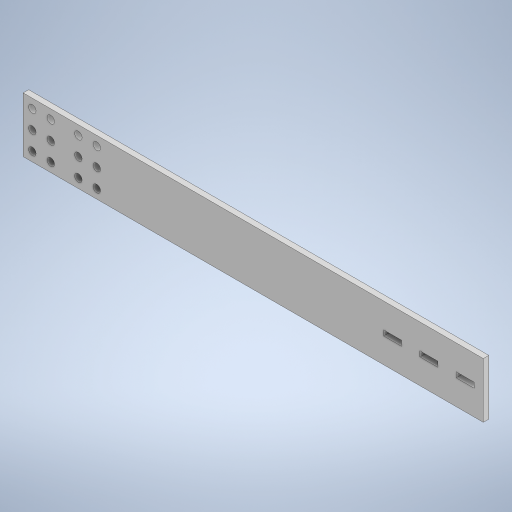
# Autodesk Inventor part: holder_sides
Saved by Autodesk Inventor 2023 (Build 270158000, 158)
## iProperties
Created: 2022-07-08
Part Number: holder_sides
Material: Generic
Document SubType Name: Modeling
Designer: Zayed
Density: 1 g/cm^3
Appearance: Default
Author: Zayed
Autodesk Inventor part; units mm, degrees
ref_plane "YZ Plane" through (0, 0, 0) normal (1, 0, 0) x (0, 1, 0)
ref_plane "XZ Plane" through (0, 0, 0) normal (0, 1, 0) x (-1, 0, 0)
ref_plane "XY Plane" through (0, 0, 0) normal (0, 0, 1) x (1, 0, 0)
sketch "Sketch1" plane through (0, 0, 0) normal (0, 0, 1) x (1, 0, 0)
  line L0 (0, 0) -> (250, 0)
  line L1 (250, 0) -> (250, 30)
  line L2 (-250, -30) -> (250, -30)
  line L3 (250, -30) -> (250, 30)
  line L4 (250, 30) -> (-250, 30)
  line L5 (-250, 30) -> (-250, -30)
  line L6 (-250, -30) -> (250, 30) construction
  line L7 (250, -30) -> (-250, 30) construction
  line L8 (-250, 0) -> (-240, 0)
  line L9 (-240, 0) -> (-240, 20)
  line L10 (-240, 0) -> (-240, -20)
  circle A0 centre (-240, 0) radius 4
  circle A1 centre (-240, 20) radius 4
  circle A2 centre (-240, -20) radius 4
  line L11 (-240, 0) -> (-220, 0)
  line L12 (-220, 0) -> (-220, -20)
  line L13 (-220, 0) -> (-220, 20)
  circle A3 centre (-220, 20) radius 4
  circle A4 centre (-220, 0) radius 4
  circle A5 centre (-220, -20) radius 4
  line L14 (-220, 0) -> (-190, 0)
  line L15 (-190, 0) -> (-190, -20)
  line L16 (-190, 0) -> (-190, 20)
  line L17 (-190, 0) -> (-170, 0)
  line L18 (-170, 0) -> (-170, -20)
  line L19 (-170, 0) -> (-170, 20)
  circle A6 centre (-190, 20) radius 4
  circle A7 centre (-170, 20) radius 4
  circle A8 centre (-170, 0) radius 4
  circle A9 centre (-170, -20) radius 4
  circle A10 centre (-190, 0) radius 4
  circle A11 centre (-190, -20) radius 4
  line L20 (250, 0) -> (240, 0)
  line L21 (240, 0) -> (230.3, 0)
  line L22 (240, 0) -> (240, 2.85)
  line L23 (220.6, -2.85) -> (240, -2.85)
  line L24 (240, -2.85) -> (240, 2.85)
  line L25 (240, 2.85) -> (220.6, 2.85)
  line L26 (220.6, 2.85) -> (220.6, -2.85)
  line L27 (220.6, -2.85) -> (240, 2.85) construction
  line L28 (240, -2.85) -> (220.6, 2.85) construction
  line L29 (220.6, 0) -> (200.6, 0)
  line L30 (200.6, 0) -> (200.6, -2.85)
  line L31 (200.6, 0) -> (190.9, 0)
  line L32 (181.2, 2.85) -> (200.6, 2.85)
  line L33 (200.6, 2.85) -> (200.6, -2.85)
  line L34 (200.6, -2.85) -> (181.2, -2.85)
  line L35 (181.2, -2.85) -> (181.2, 2.85)
  line L36 (181.2, 2.85) -> (200.6, -2.85) construction
  line L37 (200.6, 2.85) -> (181.2, -2.85) construction
  line L38 (181.2, 0) -> (161.2, 0)
  line L39 (161.2, 0) -> (161.2, -2.85)
  line L40 (161.2, 0) -> (151.5, 0)
  line L41 (141.8, 2.85) -> (161.2, 2.85)
  line L42 (161.2, 2.85) -> (161.2, -2.85)
  line L43 (161.2, -2.85) -> (141.8, -2.85)
  line L44 (141.8, -2.85) -> (141.8, 2.85)
  line L45 (141.8, 2.85) -> (161.2, -2.85) construction
  line L46 (161.2, 2.85) -> (141.8, -2.85) construction
  dimension "d0" = 250
  dimension "d1" = 30
  dimension "d2" = 10
  dimension "d3" = 20
  dimension "d4" = 20
  dimension "d5" = 8
  dimension "d6" = 8
  dimension "d7" = 8
  dimension "d8" = 20
  dimension "d9" = 8
  dimension "d10" = 8
  dimension "d11" = 8
  dimension "d12" = 30
  dimension "d13" = 20
  dimension "d14" = 8
  dimension "d15" = 8
  dimension "d16" = 8
  dimension "d17" = 8
  dimension "d18" = 8
  dimension "d19" = 8
  dimension "d20" = 10
  dimension "d21" = 9.7
  dimension "d22" = 2.85
  dimension "d25" = 20
  dimension "d26" = 9.7
  dimension "d27" = 20
  dimension "d28" = 9.7
  constraints: 94 end point, 12 centre point, 12 coincident, 11 midpoint, 9 horizontal, 8 parallel, 8 perpendicular, 8 vertical, 6 point on line
  measures "d0" distance of L0.start L0.end
  measures "d1" distance of L0.end L1.end
  measures "d2" distance of L8.start L8.end
  measures "d3" distance of L8.end L9.end
  measures "d4" distance of L8.end L10.end
  measures "d5" diameter of A0
  measures "d6" diameter of A1
  measures "d7" diameter of A2
  measures "d8" distance of L11.start L11.end
  measures "d9" diameter of A3
  measures "d10" diameter of A4
  measures "d11" diameter of A5
  measures "d12" distance of L14.start L14.end
  measures "d13" distance of L14.end L17.end
  measures "d14" diameter of A6
  measures "d15" diameter of A7
  measures "d16" diameter of A8
  measures "d17" diameter of A9
  measures "d18" diameter of A10
  measures "d19" diameter of A11
  measures "d20" distance of L0.end L20.end
  measures "d21" distance of L20.end L21.end
  measures "d22" distance of L20.end L22.end
  measures "d25" distance of L29.start L29.end
  measures "d26" distance of L29.end L31.end
  measures "d27" distance of L38.start L38.end
  measures "d28" distance of L38.end L40.end
extrude "Extrusion2" add sketch "Sketch1" along normal blind 6
body "Solid2"
